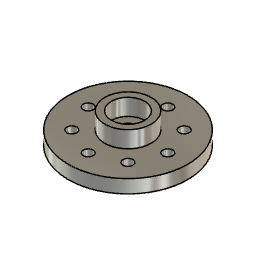
小舵机舵盘 v2 (Autodesk Fusion 360 design; units mm, degrees)
Autodesk Fusion 360 part; units mm, degrees
sketch "草图1" plane through (0, 0, 0) normal (0, 0, 1) x (1, 0, 0)
  circle A0 centre (0, 0) radius 9
  circle A1 centre (0, 0) radius 1.25
  line L0 (0, 0) -> (12.5942, 0) construction
  circle A2 centre (0, 0) radius 6 construction
  circle A3 centre (6, 0) radius 0.75
  circle A4 centre (4.2426, 4.2426) radius 0.75
  circle A5 centre (0, 6) radius 0.75
  circle A6 centre (-4.2426, 4.2426) radius 0.75
  circle A7 centre (-6, 0) radius 0.75
  circle A8 centre (-4.2426, -4.2426) radius 0.75
  circle A9 centre (0, -6) radius 0.75
  circle A10 centre (4.2426, -4.2426) radius 0.75
  dimension "d1" = 18
  dimension "d2" = 2.5
  dimension "d3" = 12
  dimension "d4" = 1.5
  dimension "d6" = 360
  constraint coincident A0.centre A1.centre
  constraint horizontal L0
  constraint concentric A0 A2
  constraint coincident A2 A3.centre
  constraint coincident L0 A3.centre
  measures "d1" diameter of A0
  measures "d2" diameter of A1
  measures "d3" diameter of A2
  measures "d4" diameter of A3
extrude "拉伸1" add sketch "草图1" along normal blind 2
sketch "草图2" plane through (0, 0, 2) normal (0, 0, 1) x (-1, 0, 0)
  circle A0 centre (6, 0) radius 0.75
  circle A1 centre (0, 6) radius 0.75
  circle A2 centre (-4.2426, -4.2426) radius 0.75
  circle A3 centre (4.2426, 4.2426) radius 0.75
  circle A4 centre (0, -6) radius 0.75
  circle A5 centre (0, 0) radius 1.25
  circle A6 centre (4.2426, -4.2426) radius 0.75
  circle A7 centre (-6, 0) radius 0.75
  circle A8 centre (-4.2426, 4.2426) radius 0.75
  circle A9 centre (0, 0) radius 9
  circle A10 centre (0, 0) radius 3.5
  circle A11 centre (0, 0) radius 2.5
  dimension "d9" = 7
  dimension "d10" = 5
  constraint concentric A5 A10
  constraint coincident A5.centre A9.centre
  measures "d9" diameter of A10
  measures "d10" diameter of A11
extrude "拉伸2" add sketch "草图2" along normal blind 2.5 contours A10
